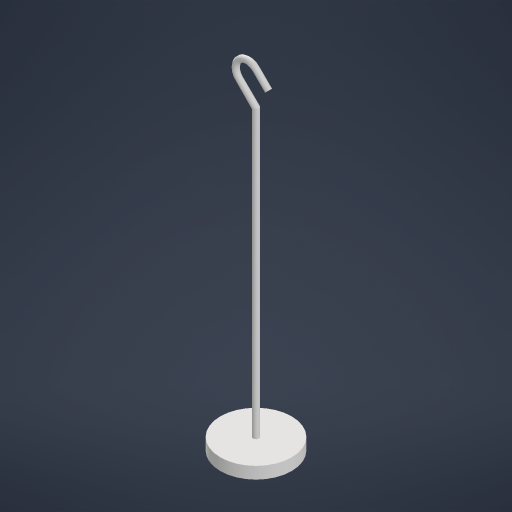
# Autodesk Inventor part: Long Hanging Mass
Saved by Autodesk Inventor 2023.1 (Build 271208000, 208)
## iProperties
Created: 2022-12-07
Part Number: Long Hanging Mass
Material: Generic
Document SubType Name: Modeling
Designer: aubrey-work
Density: 1 g/cm^3
Appearance: Default
Author: aubrey-work
Autodesk Inventor part; units mm, degrees
ref_plane "YZ Plane" through (0, 0, 0) normal (1, 0, 0) x (0, 1, 0)
ref_plane "XZ Plane" through (0, 0, 0) normal (0, 1, 0) x (-1, 0, 0)
ref_plane "XY Plane" through (0, 0, 0) normal (0, 0, 1) x (1, 0, 0)
sketch "Sketch1" plane through (0, 0, 0) normal (0, 1, 0) x (-1, 0, 0)
  circle A0 centre (0, 0) radius 19.05
  dimension "d0" = 38.1
  constraints: 1 centre point, 1 coincident
  measures "d0" diameter of A0
extrude "Extrusion1" add sketch "Sketch1" along normal blind 6.35
sketch "Sketch2" plane through (0, 0, 0) normal (0, 0, 1) x (1, 0, 0)
  line L0 (19.05, 6.35) -> (-19.05, 6.35) projected
  line L1 (0, 6.35) -> (0, 158.75)
  line L2 (0, 158.75) -> (-4.4901, 163.2401)
  line L3 (0, 158.75) -> (6.35, 158.75) construction
  circle A0 centre (-4.4901, 172.2204) radius 6.35 construction
  line L4 (-4.4901, 163.2401) -> (25.7701, 193.5003) construction
  line L5 (-4.4901, 163.2401) -> (-8.9803, 167.7303)
  line L6 (0, 176.7105) -> (6.7352, 169.9753)
  arc A1 (0, 176.7105) -> (-8.9803, 167.7303) centre (-4.4901, 172.2204) ccw
  point P0 (0, 0)
  dimension "d3" = 152.4
  dimension "d4" = 6.35
  dimension "d5" = 135
  dimension "d6" = 12.7
  dimension "d7" = 9.525
  constraints: 12 end point, 5 tangent, 4 point on circle, 2 centre point, 1 equal length, 1 horizontal, 1 midpoint, 1 parallel, 1 perpendicular, 1 vertical
  measures "d3" distance of L1.start L1.end
  measures "d4" distance of L1.end L2.end
  measures "d5" angle of L3 L2
  measures "d6" diameter of A0
  measures "d7" distance of L6.start L6.end
sketch "Sketch3" plane through (0, 6.35, 0) normal (0, 1, 0) x (1, 0, 0)
  circle A0 centre (0, 0) radius 1.5875
  dimension "d8" = 3.175
  constraints: 1 centre point, 1 coincident
  measures "d8" diameter of A0
sweep "Sweep1" add profiles "Sketch3" path "Sketch2" path curves L1 L2 L5 A1 L6
body "Solid1"
